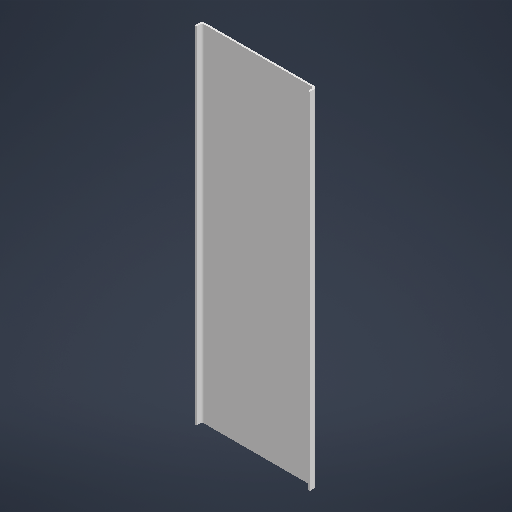
# Autodesk Inventor part: TrayRail
Saved by Autodesk Inventor 2026.3 (Build 303398000, 398)
## iProperties
Created: 2026-05-01
Part Number: TrayRail
Material: Generic
Document SubType Name: Sheet Metal
Designer: frede
Density: 1 g/cm^3
Sheet Metal Rule: Default_mm
Appearance: Default
Author: frede
Autodesk Inventor part; units mm, degrees
ref_plane "YZ Plane" through (0, 0, 0) normal (1, 0, 0) x (0, 1, 0)
ref_plane "XZ Plane" through (0, 0, 0) normal (0, 1, 0) x (-1, 0, 0)
ref_plane "XY Plane" through (0, 0, 0) normal (0, 0, 1) x (1, 0, 0)
sketch "Sketch1" plane through (0, 0, 0) normal (0, 0, 1) x (1, 0, 0)
  line L0 (61, -189) -> (-61, -189)
  line L1 (-61, -189) -> (-61, 189)
  line L2 (-61, 189) -> (61, 189)
  line L3 (61, 189) -> (61, -189)
  line L4 (61, -189) -> (-61, 189) construction
  line L5 (-61, -189) -> (61, 189) construction
  point P0 (0, 0)
  dimension "d0" = 122
  dimension "d1" = 378
  measures "d0" distance of L1.end L2.end
  measures "d1" distance between parallel lines of L0 L2
extrude "Plate1" add sketch "Sketch1" along normal blind 2
sketch "Sketch3" plane through (-63, -189, 0) normal (1, 0, 0) x (0, 1, 0)
  line L0 (378, 0) -> (0, 0)
  line L1 (0, 0) -> (0, 8)
  line L2 (0, 8) -> (378, 8)
  line L3 (378, 8) -> (378, 0)
  constraints: 8 end point
edge flange "Flange1" height 8 angle 90 thickness 2 bend radius 2 thickness toward (1, 0, 0) relief straight relief width 2 relief depth 1 corner gap 2 corner form 0 edges at (-61, 0, 2) (61, 0, 2) wall of the first edge with corners at (-63, 189, 0) (-63, -189, 0) (-63, -189, 8) (-63, 189, 8)
bend "Bend1"
corner "Corner1"
equation "\"d4\" = Thickness"
equation "\"d5\" = BendReliefWidth"
equation "\"d6\" = BendReliefDepth"
equation "\"d7\" = MinimumRemnant"
equation "\"d8\" = TransitionRadius"
equation "\"d11\" = BendRadius"
equation "\"d12\" = CornerReliefSize"
equation "\"d13\" = GapSize"
equation "\"d14\" = JacobiRadiusSize"
equation "\"BendRadius\" = Thickness"
equation "\"BendReliefWidth\" = Thickness"
equation "\"BendReliefDepth\" = 0.5 * Thickness"
equation "\"CornerReliefSize\" = 4 * Thickness"
equation "\"MinimumRemnant\" = 2 * Thickness"
equation "\"TransitionRadius\" = BendRadius"
equation "\"JacobiRadiusSize\" = BendRadius"
equation "\"GapSize\" = Thickness"
equation "\"Thickness\" = 2"
body "Solid2"
